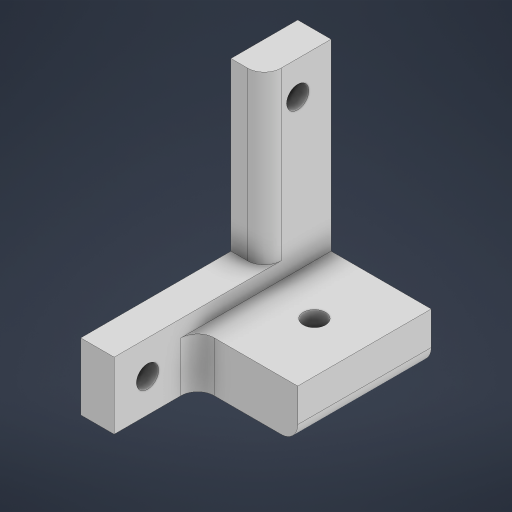
# Autodesk Inventor part: wing mount 1 v2
Saved by Autodesk Inventor 2024 (Build 280153000, 153)
## iProperties
Created: 2023-12-25
Part Number: wing mount 1 v2
Material: Generic
Document SubType Name: Modeling
Designer: elite
Density: 1 g/cm^3
Appearance: Default
Author: elite
Autodesk Inventor part; units mm, degrees
ref_plane "YZ Plane" through (0, 0, 0) normal (1, 0, 0) x (0, 1, 0)
ref_plane "XZ Plane" through (0, 0, 0) normal (0, 1, 0) x (-1, 0, 0)
ref_plane "XY Plane" through (0, 0, 0) normal (0, 0, 1) x (1, 0, 0)
sketch "Sketch1" plane through (0, 0, 0) normal (1, 0, 0) x (0, 1, 0)
  line L0 (0, 0) -> (0, -28.575)
  line L1 (0, -28.575) -> (31.75, -28.575)
  circle A0 centre (31.75, -28.575) radius 2.1082
  circle A1 centre (0, 0) radius 2.1082
  line L2 (31.75, -28.575) -> (31.75, -34.925)
  line L3 (31.75, -34.925) -> (38.1, -34.925)
  line L4 (0, 0) -> (-6.35, 0)
  line L5 (-6.35, 0) -> (-6.35, 6.35)
  line L6 (0, 0) -> (6.35, 0)
  line L7 (0, -28.575) -> (0, -34.925)
  line L8 (-6.35, 6.35) -> (6.35, 6.35)
  line L9 (6.35, 6.35) -> (6.35, -34.925)
  line L10 (6.35, -34.925) -> (-6.35, -34.925)
  line L11 (-6.35, -34.925) -> (-6.35, 6.35)
  line L12 (0, -28.575) -> (0, -22.225)
  line L13 (0, -22.225) -> (38.1, -22.225)
  line L14 (38.1, -22.225) -> (38.1, -34.925)
  line L15 (38.1, -34.925) -> (0, -34.925)
  line L16 (0, -34.925) -> (0, -22.225)
  point P0 (6.35, -22.225)
  dimension "d0" = 28.575
  dimension "d1" = 31.75
  dimension "d2" = 4.2164
  dimension "d3" = 4.2164
  dimension "d4" = 6.35
  dimension "d5" = 6.35
  dimension "d6" = 6.35
  dimension "d7" = 6.35
  dimension "d8" = 6.35
  dimension "d9" = 6.35
  dimension "d10" = 6.35
  constraints: 34 end point, 5 perpendicular, 4 horizontal, 4 parallel, 3 vertical, 2 centre point, 2 coincident, 1 point on line
  measures "d0" distance of L0.start L0.end
  measures "d1" distance of L0.end L1.end
  measures "d2" diameter of A0
  measures "d3" diameter of A1
  measures "d4" distance of L2.start L2.end
  measures "d5" distance of L2.end L3.end
  measures "d6" distance of L4.start L4.end
  measures "d7" distance of L4.end L5.end
  measures "d8" distance of L4.start L6.end
  measures "d9" distance of L0.end L7.end
  measures "d10" distance of L0.end L12.end
extrude "Extrusion1" add sketch "Sketch1" along normal blind 6.35 contours L13 L9 L1 L0 | L0 L7 L10 L11 L4 A1 | L0 A1 L6 L9 L13 | L1 L9 L10 L7 | L13 L14 L3 L2 A0 L1 L9 | L1 A0 L2 L15 L9 | L4 L5 L8 L9 L6 A1
sketch "Sketch2" plane through (6.35, 0, 0) normal (1, 0, 0) x (0, 0, -1)
  line L0 (34.925, -6.35) -> (34.925, 38.1) projected
  line L1 (22.225, 6.35) -> (-6.35, 6.35) projected
  line L2 (34.925, -6.35) -> (9.525, -6.35)
  line L3 (9.525, -6.35) -> (9.525, 6.35)
  line L4 (9.525, 6.35) -> (34.925, 6.35)
  line L5 (34.925, 6.35) -> (34.925, -6.35)
  point P0 (0, 0)
  dimension "d13" = 25.4
  constraints: 8 end point, 2 parallel, 1 horizontal, 1 perpendicular, 1 point on line
  measures "d13" distance of L3.end L4.end
extrude "Extrusion2" add sketch "Sketch2" along normal blind 19.05
fillet "Fillet1" radius 3.175 1 edges at (6.35, 22.225, -22.225)
fillet "Fillet2" radius 3.175 1 edges at (6.35, 0, -9.525)
fillet "Fillet3" radius 3.175 1 edges at (25.4, -6.35, -22.225)
sketch "Sketch3" plane through (0, 6.35, 6.35) normal (0, 1, 0) x (1, 0, 0)
  line L0 (6.35, 31.75) -> (6.35, 41.275) projected
  line L1 (6.35, 41.275) -> (28.2594, 41.275)
  line L2 (28.2594, 41.275) -> (28.2594, 9.9095)
  line L3 (28.2594, 9.9095) -> (6.35, 9.9095)
  line L4 (6.35, 9.9095) -> (6.35, 41.275)
  point P0 (0, 6.35)
  constraints: 8 end point, 2 parallel, 1 horizontal, 1 perpendicular
extrude "Extrusion3" cut sketch "Sketch3" against normal blind 3.175
sketch "Sketch4" plane through (0, 3.175, 6.35) normal (0, 1, 0) x (1, 0, 0)
  line L0 (6.35, 12.7) -> (6.35, 41.275) projected
  line L1 (6.35, 41.275) -> (25.4, 15.875)
  circle A0 centre (15.875, 28.575) radius 2.1082
  point P0 (0, 6.35)
  dimension "d21" = 4.2164
  constraints: 2 end point, 1 centre point, 1 midpoint
  measures "d21" diameter of A0
extrude "Extrusion4" cut sketch "Sketch4" against normal blind 20.6375
body "Solid1"
